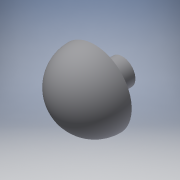
# Autodesk Inventor part: slider
Saved by Autodesk Inventor 2017 (Build 210142000, 142)
## iProperties
Created: 2018-04-19
Part Number: slider
Material: Generic
Document SubType Name: Modeling
Designer: winda
Density: 1 g/cm^3
Appearance: Default
Author: winda
Autodesk Inventor part; units mm, degrees
ref_plane "YZ Plane" through (0, 0, 0) normal (1, 0, 0) x (0, 1, 0)
ref_plane "XZ Plane" through (0, 0, 0) normal (0, 1, 0) x (-1, 0, 0)
ref_plane "XY Plane" through (0, 0, 0) normal (0, 0, 1) x (1, 0, 0)
sketch "Sketch1" plane through (0, 0, 0) normal (0, 0, 1) x (1, 0, 0)
  arc A0 (-4, 0) -> (4, 0) centre (0, 0) ccw
  line L0 (-4, 0) -> (0, 0)
  line L1 (0, 0) -> (4, 0)
  line L2 (-1.4, 0) -> (-1.4, 3)
  line L3 (-1.4, 3) -> (1.4, 3)
  line L4 (1.4, 3) -> (1.4, 0)
  line L5 (0, 6.1) -> (0, -11.2301) construction
  line L6 (0, 3) -> (0, 0)
  line L7 (0, 0) -> (0, -4)
  dimension "d0" = 8
  dimension "d1" = 1.4
  dimension "d2" = 1.4
  dimension "d3" = 3
  constraints: 16 end point, 5 point on line, 3 perpendicular, 3 point on circle, 2 vertical, 1 centre point, 1 coincident, 1 horizontal, 1 midpoint
  measures "d0" diameter of A0
  measures "d1" distance from line of L4 point (0, 0)
  measures "d2" distance from line of L2 point (0, 0)
  measures "d3" distance from line of point (0, 0) L3
revolve "Revolution1" add sketch "Sketch1" angle 360 about axis through (0, 6.1, 0) along (0, -1, 0) contours L0 L7 A0 | L2 L3 L6 L0
body "Solid1"
